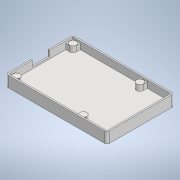
# Autodesk Inventor part: Pi Back Mount
Saved by Autodesk Inventor 2020.3 (Build 243373010, 373A)
## iProperties
Created: 2021-08-29
Part Number: Pi Back Mount
Material: Generic
Document SubType Name: Modeling
Designer: Parker
Density: 1 g/cm^3
Appearance: Default
Author: Parker
Autodesk Inventor part; units mm, degrees
ref_plane "YZ Plane" through (0, 0, 0) normal (1, 0, 0) x (0, 1, 0)
ref_plane "XZ Plane" through (0, 0, 0) normal (0, 1, 0) x (-1, 0, 0)
ref_plane "XY Plane" through (0, 0, 0) normal (0, 0, 1) x (1, 0, 0)
sketch "Sketch1" plane through (0, 0, 0) normal (0, 1, 0) x (-1, 0, 0)
  line L0 (29, 24.5) -> (-29, 24.5) construction
  line L1 (-29, 24.5) -> (-29, -24.5) construction
  line L2 (-29, -24.5) -> (29, -24.5) construction
  line L3 (29, -24.5) -> (29, 24.5) construction
  circle A0 centre (29, 24.5) radius 3
  circle A1 centre (29, -24.5) radius 3
  circle A2 centre (-29, -24.5) radius 3
  circle A3 centre (-29, 24.5) radius 3
  point P0 (0, 0)
  dimension "d0" = 24.5
  dimension "d1" = 29
  dimension "d2" = 58
  dimension "d3" = 49
  dimension "d4" = 6
  dimension "d5" = 6
  dimension "d6" = 6
  dimension "d7" = 6
  constraints: 8 coincident, 8 end point, 4 centre point, 2 parallel, 1 horizontal, 1 perpendicular
  measures "d0" vertical distance of point (0, 0) L0.start
  measures "d1" horizontal distance of point (0, 0) L0.start
  measures "d2" distance of L2.end L1.end
  measures "d3" distance of L1.end L0.end
  measures "d4" diameter of A0
  measures "d5" diameter of A1
  measures "d6" diameter of A2
  measures "d7" diameter of A3
extrude "Extrusion1" add sketch "Sketch1" along normal blind 5
sketch "Sketch6" plane through (0, 0, 0) normal (0, 1, 0) x (-1, 0, 0)
  line L0 (33.8, -29.3) -> (-55, -29.3)
  line L1 (-55, -29.3) -> (-55, 29.3)
  line L2 (-55, 29.3) -> (33.8, 29.3)
  line L3 (33.8, 29.3) -> (33.8, -29.3)
  circle A0 centre (29, -24.5) radius 3 projected
  circle A1 centre (-29, 24.5) radius 3 projected
  circle A2 centre (29, 24.5) radius 3 projected
  circle A3 centre (-29, -24.5) radius 3 projected
  line L4 (32, -27.5) -> (-32, -27.5)
  line L5 (-32, -27.5) -> (-32, 27.5)
  line L6 (-32, 27.5) -> (32, 27.5)
  line L7 (32, 27.5) -> (32, -27.5)
  point P0 (0, 0)
  dimension "d30" = 1.8
  dimension "d31" = 55
  dimension "d32" = 64
  dimension "d33" = 27.5
  dimension "d34" = 32
  dimension "d35" = 1.8
  dimension "d36" = 1.8
  dimension "d37" = 23
  constraints: 16 end point, 4 parallel, 2 horizontal, 2 perpendicular
  measures "d30" distance between parallel lines of L3 L7
  measures "d31" distance of L6.end L4.start
  measures "d32" distance of L4.start L4.end
  measures "d33" distance from line of point (0, 0) L4
  measures "d34" distance from line of L7 point (0, 0)
  measures "d35" distance between parallel lines of L4 L0
  measures "d36" distance between parallel lines of L2 L6
  measures "d37" distance between parallel lines of L5 L1
extrude "Extrusion5" add sketch "Sketch6" against normal blind 3 contours L0 L1 L2 L3 | A0 | L7 L4 A0 | A0 L4 A3 L5 A1 L6 A2 L7 | A2 | A2 L6 L7 | L4 L5 A3 | A3 | A1 | A1 L5 L6
fillet "Fillet2" radius 2 4 edges at (-33.8, -1.5, 29.3) (55, -1.5, 29.3) (55, -1.5, -29.3) (-33.8, -1.5, -29.3)
sketch "Sketch7" plane through (0, 0, 0) normal (0, 1, 0) x (1, 0, 0)
  circle A0 centre (29, 24.5) radius 3 projected
  circle A1 centre (-29, 24.5) radius 3 projected
  circle A2 centre (29, -24.5) radius 3 projected
  circle A3 centre (-29, -24.5) radius 3 projected
  arc A4 (-31.8, 29.3) -> (-33.8, 27.3) centre (-31.8, 27.3) ccw projected
  line L0 (-33.8, 27.3) -> (-33.8, -27.3) projected
  arc A5 (-33.8, -27.3) -> (-31.8, -29.3) centre (-31.8, -27.3) ccw projected
  line L1 (-31.8, -29.3) -> (53, -29.3) projected
  arc A6 (53, -29.3) -> (55, -27.3) centre (53, -27.3) ccw projected
  line L2 (55, -27.3) -> (55, 27.3) projected
  arc A7 (55, 27.3) -> (53, 29.3) centre (53, 27.3) ccw projected
  line L3 (53, 29.3) -> (-31.8, 29.3) projected
  line L4 (53.8, 27.3) -> (53.8, -27.3)
  arc A8 (53, -28.1) -> (53.8, -27.3) centre (53, -27.3) ccw
  line L5 (53, -28.1) -> (-31.8, -28.1)
  arc A9 (-32.6, -27.3) -> (-31.8, -28.1) centre (-31.8, -27.3) ccw
  line L6 (-32.6, -27.3) -> (-32.6, 27.3)
  arc A10 (-31.8, 28.1) -> (-32.6, 27.3) centre (-31.8, 27.3) ccw
  line L7 (-31.8, 28.1) -> (53, 28.1)
  arc A11 (53.8, 27.3) -> (53, 28.1) centre (53, 27.3) ccw
  point P0 (0, 0)
  dimension "d41" = 1.2
  constraints: 8 end point, 8 point on circle, 4 centre point, 7 other
  measures "d41" distance between parallel lines of L2 L4
extrude "Extrusion6" add sketch "Sketch7" along normal blind 6.5 contours L3 A7 L2 A6 L1 A5 L0 A4
sketch "Sketch8" plane through (0, 0, 0) normal (0, 1, 0) x (1, 0, 0)
  arc A0 (-31.8, 28.1) -> (-32.6, 27.3) centre (-31.8, 27.3) ccw projected
  line L0 (-32.6, 27.3) -> (-32.6, -27.3) projected
  arc A1 (-32.6, -27.3) -> (-31.8, -28.1) centre (-31.8, -27.3) ccw projected
  line L1 (-31.8, -28.1) -> (53, -28.1) projected
  arc A2 (53, -28.1) -> (53.8, -27.3) centre (53, -27.3) ccw projected
  line L2 (53.8, -27.3) -> (53.8, 27.3) projected
  arc A3 (53.8, 27.3) -> (53, 28.1) centre (53, 27.3) ccw projected
  line L3 (53, 28.1) -> (-31.8, 28.1) projected
  circle A4 centre (29, 24.5) radius 3 projected
  circle A5 centre (-29, 24.5) radius 3 projected
  circle A6 centre (29, -24.5) radius 3 projected
  circle A7 centre (-29, -24.5) radius 3 projected
  circle A8 centre (-29, -24.5) radius 3 projected
  line L4 (-29, -21.5) -> (-32.6, -21.5)
  line L5 (-32.6, 27.3) -> (-32.6, -27.3) projected
  line L6 (-26, -24.5) -> (-26, -28.1)
  line L7 (-31.8, -28.1) -> (53, -28.1) projected
  circle A9 centre (-29, 24.5) radius 3 projected
  line L8 (-29, 21.5) -> (-32.6, 21.5)
  line L9 (-26, 24.5) -> (-26, 28.1)
  line L10 (53, 28.1) -> (-31.8, 28.1) projected
  circle A10 centre (29, 24.5) radius 3 projected
  line L11 (26, 24.5) -> (26, 28.1)
  line L12 (32, 24.5) -> (32, 28.1)
  circle A11 centre (29, -24.5) radius 3 projected
  line L13 (32, -24.5) -> (32, -28.1)
  line L14 (26, -24.5) -> (26, -28.1)
  point P0 (0, 0)
  constraints: 16 end point, 14 point on line, 5 perpendicular, 4 point on circle, 4 tangent, 1 horizontal alignment, 1 vertical alignment, 6 other
extrude "Extrusion7" add sketch "Sketch8" along normal blind 4.8 contours L3 L9 A5 L8 L0 A0 | L3 L12 A4 L11 | L4 A7 L6 L1 A1 L0 | L14 A6 L13 L1
sketch "Sketch9" plane through (-33.8, -3, -27.3) normal (-1, 0, 0) x (0, 0, 1)
  line L0 (0, 0) -> (0, 9.5) projected
  line L1 (54.6, 0) -> (0, 0) projected
  line L2 (54.6, 9.5) -> (54.6, 0) projected
  line L3 (0, 9.5) -> (54.6, 9.5) projected
  line L4 (19.8, 14.5) -> (34.8, 14.5)
  line L5 (34.8, 14.5) -> (34.8, 4.5)
  line L6 (34.8, 4.5) -> (19.8, 4.5)
  line L7 (19.8, 4.5) -> (19.8, 14.5)
  line L8 (0, 9.5) -> (54.6, 9.5) projected
  line L9 (19.8, 14.5) -> (34.8, 4.5) construction
  line L10 (34.8, 14.5) -> (19.8, 4.5) construction
  point P0 (27.3, 3)
  point P1 (27.3, 9.5)
  point P2 (34.8, 9.5)
  point P3 (19.8, 9.5)
  dimension "d46" = 15
  dimension "d47" = 10
  constraints: 12 end point, 3 midpoint, 2 parallel, 1 horizontal, 1 perpendicular
  measures "d46" distance of L5.end L6.end
  measures "d47" distance of L4.end L5.end
extrude "Extrusion8" cut sketch "Sketch9" against normal up to next contours L3 L5 L6 L7
sketch "Sketch10" plane through (-29, 5, 24.5) normal (0, 1, 0) x (1, 0, 0)
  circle A0 centre (0, 0) radius 3 projected
  circle A1 centre (0, 49) radius 3 projected
  circle A2 centre (58, 49) radius 3 projected
  circle A3 centre (58, 0) radius 3 projected
  point P0 (29, 24.5)
hole "Hole2" at (-29, 5, 24.5) at (-29, 5, -24.5) at (29, 5, -24.5) at (29, 5, 24.5) direction (0, -1, 0) diameter 3.3 end through all
body "Solid1"
